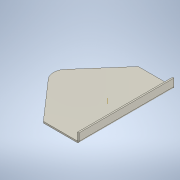
# Autodesk Inventor part: Base Plate
Saved by Autodesk Inventor 2022 (Build 260153000, 153)
## iProperties
Created: 2022-08-09
Part Number: Base Plate
Material: Steel, Galvanneal, A653 1010
Document SubType Name: Sheet Metal
Designer: Nick
Density: 7.86 g/cm^3
Appearance: Steel - Cast
Sheet Metal Rule: STL A653 1010 Galvanneal .093 (13ga)
Mass: 92.5141 g
Surface Area: 453.074 cm^2
Volume: 51.4197 cm^3
Author: Nick
Autodesk Inventor part; units mm, degrees
ref_plane "YZ Plane" through (0, 0, 0) normal (1, 0, 0) x (0, 1, 0)
ref_plane "XZ Plane" through (0, 0, 0) normal (0, 1, 0) x (-1, 0, 0)
ref_plane "XY Plane" through (0, 0, 0) normal (0, 0, 1) x (1, 0, 0)
sketch "Sketch1" plane through (0, 0, 0) normal (0, 1, 0) x (-1, 0, 0)
  line L0 (0, 0) -> (55, 0)
  line L1 (55, 0) -> (55, -152.4)
  line L2 (55, -152.4) -> (0, -152.4)
  line L3 (0, -152.4) -> (0, 0)
  dimension "d0" = 55
  dimension "d1" = 152.4
  measures "d0" distance of L1.end L2.end
  measures "d1" distance of L0.end L1.end
ref_plane "Work Plane1" through (-55, 0, -76.2) normal (0, 0, 1) x (1, 0, 0)
ref_plane "Work Plane2" through (-27.5, 0, 0) normal (1, 0, 0) x (0, 0, -1)
sketch "Sketch2" plane through (0, 2.3622, 0) normal (0, 1, 0) x (1, 0, 0)
  line L0 (-55, 0) -> (-55, 152.4)
  line L1 (-55, 0) -> (-110.0633, 63.0434)
  line L2 (-110.0633, 89.3566) -> (-55, 152.4)
  arc A0 (-110.0633, 89.3566) -> (-110.0633, 63.0434) centre (-95, 76.2) ccw
  line L3 (0, 0) -> (-55, 0)
  point P0 (-55, 76.2)
  dimension "d3" = 20
  dimension "d4" = 40
  measures "d3" radius of A0
  measures "d4" distance from line of L0 A0.centre
extrude "Plate1" add sketch "Sketch1" along normal blind 2.3622
sheet face with bend "Face2" sketch "Sketch2" thickness 2.3622 toward (0, -1, 0) bend radius 0.7937 relief straight relief width 2.3622 relief depth 1.1811
bend "Bend1"
sketch "Sketch3" plane through (0, 2.3622, -152.4) normal (1, 0, 0) x (0, 1, 0)
  line L0 (0, 152.4) -> (0, 0)
  line L1 (0, 0) -> (12.6378, 0)
  line L2 (12.6378, 0) -> (12.6378, 152.4)
  line L3 (12.6378, 152.4) -> (0, 152.4)
  constraints: 6 end point, 1 horizontal, 1 perpendicular, 1 vertical
edge flange "Flange1" height 15 angle 90 thickness 2.3622 bend radius 0.7937 thickness toward (1, 0, 0) relief straight relief width 2.3622 relief depth 1.1811 edges at (0, 2.3622, -76.2) wall of the first edge with corners at (0, 2.3622, 0) (0, 2.3622, -152.4) (0, 15, -152.4) (0, 15, 0)
bend "Bend2"
corner "Corner1"
equation "\"d2\" = Thickness"
equation "\"d6\" = BendRadius"
equation "\"d7\" = BendReliefWidth"
equation "\"d9\" = MinimumRemnant"
equation "\"d8\" = BendReliefDepth"
equation "\"d10\" = TransitionRadius"
equation "\"d11\" = BendReliefWidth"
equation "\"d12\" = BendReliefDepth"
equation "\"d13\" = MinimumRemnant"
equation "\"d14\" = TransitionRadius"
equation "\"d17\" = BendRadius"
equation "\"d18\" = CornerReliefSize"
equation "\"d19\" = GapSize"
equation "\"d20\" = JacobiRadiusSize"
equation "\"BendReliefWidth\" = Thickness"
equation "\"BendReliefDepth\" = 0.5 * Thickness"
equation "\"CornerReliefSize\" = 3 * Thickness"
equation "\"MinimumRemnant\" = 2 * Thickness"
equation "\"TransitionRadius\" = BendRadius"
equation "\"JacobiRadiusSize\" = BendRadius"
equation "\"GapSize\" = 0.5 * Thickness"
equation "\"Thickness\" = 2.3622"
equation "\"BendRadius\" = 0.79375"
body "Solid1"
